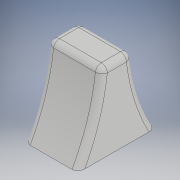
# Autodesk Inventor part: SingleSliderCap
Saved by Autodesk Inventor 2018.3 (Build 223284000, 284)
## iProperties
Created: 2019-03-27
Part Number: SingleSliderCap
Material: Generic
Document SubType Name: Modeling
Designer: matth
Density: 1 g/cm^3
Appearance: Default
Author: matth
Autodesk Inventor part; units mm, degrees
ref_plane "YZ Plane" through (0, 0, 0) normal (1, 0, 0) x (0, 1, 0)
ref_plane "XZ Plane" through (0, 0, 0) normal (0, 1, 0) x (-1, 0, 0)
ref_plane "XY Plane" through (0, 0, 0) normal (0, 0, 1) x (1, 0, 0)
sketch "Sketch1" plane through (0, 0, 0) normal (0, 0, 1) x (1, 0, 0)
  line L0 (-5.7947, 5.8302) -> (7.2053, 5.8302)
  line L1 (7.2053, 5.8302) -> (7.2053, -7.1698)
  line L2 (7.2053, -7.1698) -> (-5.7947, -7.1698)
  line L3 (-5.7947, -7.1698) -> (-5.7947, 5.8302)
  arc A0 (-5.7947, -7.1698) -> (-1.7947, 5.8302) centre (-34.6583, 8.8267) ccw
  arc A1 (3.2053, 5.8302) -> (7.2053, -7.1698) centre (36.069, 8.8267) ccw
  point P0 (0, 0)
  dimension "d0" = 13
  dimension "d1" = 13
  dimension "d2" = 4
  dimension "d3" = 4
  dimension "d4" = 33
  dimension "d5" = 33
  constraints: 8 end point, 4 point on circle, 2 centre point, 2 parallel, 2 point on line, 1 horizontal, 1 perpendicular
  measures "d0" distance of L1.end L2.end
  measures "d1" distance of L0.end L1.end
  measures "d2" distance from line of L3 A0.end
  measures "d3" distance from line of L1 A1.start
  measures "d4" radius of A0
  measures "d5" radius of A1
extrude "Extrusion1" add sketch "Sketch1" along normal blind 8.976 contours L0 A1 L2 A0
sketch "Sketch2" plane through (-5.7947, -7.1698, 0) normal (0, -1, 0) x (1, 0, 0)
  line L0 (9.1, 5.238) -> (3.7, 5.238)
  line L1 (3.7, 5.238) -> (3.7, 3.738)
  line L2 (3.7, 3.738) -> (9.1, 3.738)
  line L3 (9.1, 3.738) -> (9.1, 5.238)
  line L4 (0, 8.976) -> (13, 8.976) projected
  line L5 (13, 0) -> (13, 8.976) projected
  point P0 (5.7947, 0)
  dimension "d8" = 1.5
  dimension "d9" = 5.4
  dimension "d10" = 3.738
  dimension "d11" = 3.9
  constraints: 8 end point, 2 parallel, 1 horizontal, 1 perpendicular
  measures "d8" distance of L0.end L1.end
  measures "d9" distance of L1.end L2.end
  measures "d10" distance between parallel lines of L4 L0
  measures "d11" distance between parallel lines of L5 L3
extrude "Extrusion2" cut sketch "Sketch2" against normal blind 2
sketch "Sketch3" plane through (-5.7947, -5.1698, 0) normal (0, -1, 0) x (1, 0, 0)
  line L0 (9.1, 3.738) -> (3.7, 3.738) projected
  line L1 (4, 5.238) -> (8.8, 5.238)
  line L2 (8.8, 5.238) -> (8.8, 3.738)
  line L3 (8.8, 3.738) -> (4, 3.738)
  line L4 (4, 3.738) -> (4, 5.238)
  line L5 (3.7, 5.238) -> (9.1, 5.238) projected
  line L6 (3.7, 3.738) -> (3.7, 5.238) projected
  line L7 (9.1, 5.238) -> (9.1, 3.738) projected
  point P0 (5.7947, 0)
  dimension "d14" = 0
  dimension "d15" = 0.3
  dimension "d16" = 0.3
  constraints: 8 end point, 2 parallel, 1 horizontal, 1 perpendicular, 1 point on line
  measures "d14" distance between parallel lines of L5 L1
  measures "d15" distance between parallel lines of L4 L6
  measures "d16" distance between parallel lines of L7 L2
extrude "Extrusion3" cut sketch "Sketch3" against normal blind 10 contours L0 L4 L1 L2
fillet "Fillet1" radius 1 8 edges at (3.2053, 5.8302, 4.488) (-3.1176, -0.8781, 8.976) (0.7053, 5.8302, 8.976) (-1.7947, 5.8302, 4.488) (0.7053, 5.8302, 0) (4.5283, -0.8781, 0) (-3.1176, -0.8781, 0) (4.5283, -0.8781, 8.976)
body "Solid1"
